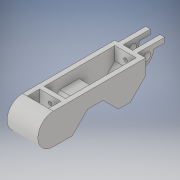
# Autodesk Inventor part: middle
Saved by Autodesk Inventor 2019 (Build 230136000, 136)
## iProperties
Created: 2018-10-13
Part Number: middle
Material: Generic
Document SubType Name: Modeling
Designer: jerem
Density: 1 g/cm^3
Appearance: Default
Author: jerem
Autodesk Inventor part; units mm, degrees
ref_plane "YZ Plane" through (0, 0, 0) normal (1, 0, 0) x (0, 1, 0)
ref_plane "XZ Plane" through (0, 0, 0) normal (0, 1, 0) x (-1, 0, 0)
sketch "Sketch2" plane through (0, 0, 0) normal (1, 0, 0) x (0, 1, 0)
  line L0 (0, 0) -> (0, -8)
  line L1 (13, 0) -> (13, -21)
  arc A0 (13, 0) -> (0, 0) centre (6.5, 0) ccw
  line L2 (-3.1385, 0) -> (18.8309, 0) projected
  line L3 (0, -58.4723) -> (0, 17.3287) projected
  line L4 (0, -8) -> (6.5, -14.5)
  line L5 (0, -8) -> (9.1924, -8) construction
  line L6 (6.5, -14.5) -> (6.5, -21)
  line L7 (6.5, -21) -> (0, -27.5)
  line L8 (6.5, -21) -> (15.6924, -21) construction
  line L9 (0, -27.5) -> (0, -32.5)
  line L10 (0, -32.5) -> (6.5, -39)
  line L11 (0, -32.5) -> (9.1924, -32.5) construction
  line L12 (13, -21) -> (13, -39)
  line L13 (13, -39) -> (13, -45.5)
  arc A1 (6.5, -39) -> (13, -45.5) centre (11.1419, -40.8581) ccw
  circle A2 centre (9.75, -43) radius 1.625
  dimension "d49" = 4
  dimension "d4" = 13
  dimension "d9" = 45
  dimension "d10" = 6.5
  dimension "d11" = 8
  dimension "d12" = 6.5
  dimension "d13" = 135
  dimension "d14" = 6.5
  dimension "d15" = 5
  dimension "d16" = 45
  dimension "d17" = 6.5
  dimension "d18" = 18
  dimension "d19" = 6.5
  dimension "d20" = 5
  dimension "d21" = 3.25
  dimension "d22" = 3.25
  dimension "d23" = 2.5
  dimension "d94" = 21
  constraints: 24 end point, 5 vertical, 4 point on circle, 3 centre point, 3 equal length, 3 horizontal, 2 point on line, 2 tangent, 1 collinear
  measures "d4" distance between parallel lines of L1 L0
  measures "d9" angle of L4 L5
  measures "d10" horizontal distance of L4.end L0.end
  measures "d11" distance of L0.start L0.end
  measures "d12" distance of L4.end L6.end
  measures "d13" angle of L7 L8
  measures "d14" horizontal distance of L7.end L6.end
  measures "d15" distance of L7.end L9.end
  measures "d16" angle of L10 L11
  measures "d17" horizontal distance of L10.end L9.end
  measures "d18" distance of L1.end L12.end
  measures "d19" distance of L12.end L13.end
  measures "d20" radius of A1
  measures "d21" diameter of A2
  measures "d22" horizontal distance of A2.centre L13.end
  measures "d23" vertical distance of L13.end A2.centre
  measures "d94" distance of L1.start L1.end
extrude "Extrusion1" add sketch "Sketch2" along normal mid plane 13 contours L2 L1 L12 L13 A1 L10 L3 L7 L6 L4 L0 | A0 L2
sketch "Sketch3" plane through (-6.5, 13, 0) normal (0, 1, 0) x (1, 0, 0)
  line L0 (0, 39) -> (13, 39) projected
  line L1 (0, 46) -> (1.5, 46)
  line L2 (1.5, 46) -> (1.5, 39)
  line L3 (1.5, 39) -> (0, 39)
  line L4 (0, 39) -> (0, 46)
  line L5 (0, 0) -> (0, 45.5) projected
  line L6 (3.5, 46) -> (7.5, 46)
  line L7 (7.5, 46) -> (7.5, 39)
  line L8 (7.5, 39) -> (3.5, 39)
  line L9 (3.5, 39) -> (3.5, 46)
  line L10 (9.5, 46) -> (13, 46)
  line L11 (13, 46) -> (13, 39)
  line L12 (13, 39) -> (9.5, 39)
  line L13 (9.5, 39) -> (9.5, 46)
  line L14 (13, 45.5) -> (13, 0) projected
  point P0 (6.5, 0)
  dimension "d47" = 1.5
  dimension "d48" = 7
  dimension "d49" = 4
  dimension "d50" = 7
  dimension "d51" = 2
  dimension "d52" = 7
  dimension "d53" = 2
  constraints: 24 end point, 6 parallel, 5 collinear, 3 horizontal, 3 perpendicular
  measures "d47" distance of L2.end L3.end
  measures "d48" distance of L1.end L2.end
  measures "d49" distance of L7.end L8.end
  measures "d50" distance of L6.end L7.end
  measures "d51" distance between parallel lines of L2 L9
  measures "d52" distance of L10.end L11.end
  measures "d53" distance between parallel lines of L13 L7
extrude "Extrusion2" cut sketch "Sketch3" against normal blind 13
ref_plane "Work Plane1" through (4.5, 0, 0) normal (1, 0, 0) x (0, 0, -1)
sketch "Sketch4" plane through (4.5, 0, 0) normal (1, 0, 0) x (0, 0, -1)
  arc A0 (0, 13) -> (0, 0) centre (0, 6.5) ccw projected
  line L0 (0, 13) -> (39, 13) projected
  line L1 (39, 13) -> (39, 6.5) projected
  line L2 (39, 6.5) -> (32.5, 0) projected
  line L3 (32.5, 0) -> (27.5, 0) projected
  line L4 (27.5, 0) -> (21, 6.5) projected
  line L5 (39, 13) -> (39, 6.5) projected
  line L6 (39, 6.5) -> (32.5, 0) projected
  line L7 (32.5, 0) -> (27.5, 0) projected
  line L8 (27.5, 0) -> (21, 6.5) projected
  line L9 (21, 6.5) -> (14.5, 6.5) projected
  line L10 (14.5, 6.5) -> (8, 0) projected
  line L11 (8, 0) -> (0, 0) projected
  arc A1 (0, 13) -> (0, 0) centre (0, 6.5) ccw projected
  line L12 (0, 13) -> (39, 13) projected
  line L13 (0, 13) -> (0, 2)
  line L14 (0, 2) -> (5.1716, 2)
  line L15 (7.1716, 2) -> (13.6716, 8.5)
  line L16 (7.1716, 2) -> (16.364, 2) construction
  line L17 (37, 13) -> (37, 7.3284)
  line L18 (37, 7.3284) -> (31.6716, 2)
  line L19 (37, 7.3284) -> (44.5355, 7.3284) construction
  line L20 (31.6716, 2) -> (28.3284, 2)
  line L21 (28.3284, 2) -> (21.8284, 8.5)
  line L22 (28.3284, 2) -> (37.5208, 2) construction
  line L23 (21.8284, 8.5) -> (13.6716, 8.5)
  line L24 (7.1716, 2) -> (7.1716, 13)
  line L25 (5.1716, 2) -> (5.1716, 13)
  line L26 (0, 13) -> (5.1716, 13)
  line L27 (7.1716, 13) -> (37, 13)
  dimension "d57" = 11
  dimension "d58" = 2
  dimension "d59" = 45
  dimension "d60" = 2
  dimension "d62" = 2
  dimension "d63" = 2
  dimension "d64" = 135
  dimension "d65" = 2
  dimension "d66" = 2
  dimension "d67" = 135
  dimension "d95" = 2
  dimension "d96" = 2
  constraints: 30 end point, 6 horizontal, 3 equal length, 3 perpendicular, 2 collinear, 1 point on line, 1 vertical
  measures "d57" distance of L12.start L13.end
  measures "d58" distance from line of L10 L15.start
  measures "d59" angle of L16 L15
  measures "d60" vertical distance of L9.end L15.end
  measures "d62" distance between parallel lines of L1 L17
  measures "d63" distance from line of L2 L17.end
  measures "d64" angle of L18 L19
  measures "d65" distance from line of L3 L18.end
  measures "d66" distance from line of L4 L20.end
  measures "d67" angle of L22 L21
  measures "d95" distance from line of L11 L15.start
  measures "d96" distance between parallel lines of L24 L25
extrude "Extrusion3" cut sketch "Sketch4" against normal blind 9 contours L0 L25 L14 L13 | L0 L17 L18 L20 L21 L23 L15 L24
sketch "Sketch5" plane through (4.5, 2, -7.1716) normal (0, 0, -1) x (-1, 0, 0)
  line L0 (0, 11) -> (0, 1) projected
  line L1 (9, 1) -> (9, 11) projected
  line L2 (0, 11) -> (0, 0) projected
  line L3 (9, 0) -> (9, 11) projected
  line L4 (0, 11) -> (9, 11) projected
  circle A0 centre (4.5, 8) radius 0.75
  circle A1 centre (4.5, 3) radius 0.75
  line L5 (0, 0) -> (9, 0) projected
  point P0 (4.5, -2)
  dimension "d72" = 1.5
  dimension "d73" = 4.5
  dimension "d74" = 3
  dimension "d75" = 1.5
  dimension "d77" = 4.5
  constraints: 2 centre point
  measures "d72" diameter of A0
  measures "d73" distance from line of L1 A0.centre
  measures "d74" distance from line of L4 A0.centre
  measures "d75" diameter of A1
  measures "d77" distance from line of L1 A1.centre
extrude "Extrusion4" cut sketch "Sketch5" against normal blind 2 contours A0 | A1
sketch "Sketch6" plane through (1, 13, -39) normal (0, 0, -1) x (-1, 0, 0)
  line L0 (1, -15.6) -> (1, 2.6) projected
  line L1 (10.1, -13) -> (-8.1, -13) projected
  circle A0 centre (1, -3) radius 0.75
  line L2 (0, 0) -> (4, 0) projected
  circle A1 centre (1, -10) radius 0.75
  point P0 (1, -13)
  dimension "d80" = 1.5
  dimension "d81" = 3
  dimension "d82" = 1.5
  dimension "d83" = 3
  constraints: 2 centre point, 2 point on line
  measures "d80" diameter of A0
  measures "d81" distance from line of L2 A0.centre
  measures "d82" diameter of A1
  measures "d83" distance from line of L1 A1.centre
extrude "Extrusion5" cut sketch "Sketch6" against normal blind 9
sketch "Sketch7" plane through (3, 13, -39) normal (1, 0, 0) x (0, 0, -1)
  line L0 (6.5, 0) -> (0, 0) projected
  line L1 (6.5, 0) -> (11.5, 0)
  line L2 (11.5, 0) -> (11.5, -2)
  line L3 (11.5, -2) -> (6.5, -2)
  line L4 (6.5, -2) -> (6.5, 0)
  point P0 (-39, -13)
  dimension "d86" = 5
  dimension "d87" = 2
  constraints: 8 end point, 2 parallel, 1 collinear, 1 horizontal, 1 perpendicular
  measures "d86" distance of L2.end L3.end
  measures "d87" distance of L1.end L2.end
extrude "Extrusion6" add sketch "Sketch7" against normal blind 2
sketch "Sketch8" plane through (-5, 13, -45.5) normal (-1, 0, 0) x (0, 0, 1)
  line L0 (0, 0) -> (6.5, 0) projected
  line L1 (-5, -2) -> (0, -2)
  line L2 (0, -2) -> (0, 0)
  line L3 (0, 0) -> (-5, 0)
  line L4 (-5, 0) -> (-5, -2)
  point P0 (45.5, -13)
  dimension "d90" = 5
  dimension "d91" = 2
  constraints: 8 end point, 2 parallel, 1 horizontal, 1 perpendicular
  measures "d90" distance of L0.start L3.end
  measures "d91" distance of L0.start L1.end
extrude "Extrusion7" add sketch "Sketch8" against normal blind 2
body "Solid1"
